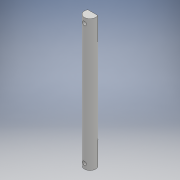
# Autodesk Inventor part: Rear Axle
Saved by Autodesk Inventor 2018 (Build 220112000, 112)
## iProperties
Created: 2018-01-31
Part Number: Rear Axle
Material: Generic
Document SubType Name: Modeling
Designer: alber
Density: 1 g/cm^3
Appearance: Default
Author: alber
Autodesk Inventor part; units mm, degrees
ref_plane "YZ Plane" through (0, 0, 0) normal (1, 0, 0) x (0, 1, 0)
ref_plane "XZ Plane" through (0, 0, 0) normal (0, 1, 0) x (-1, 0, 0)
ref_plane "XY Plane" through (0, 0, 0) normal (0, 0, 1) x (1, 0, 0)
sketch "Sketch1" plane through (0, 0, 0) normal (0, 0, 1) x (1, 0, 0)
  circle A0 centre (0, 0) radius 3.6
  dimension "d0" = 7.2
  constraints: 1 centre point, 1 coincident
  measures "d0" diameter of A0
extrude "Extrusion1" add sketch "Sketch1" along normal mid plane 83.2
sketch "Sketch2" plane through (0, 0, 41.6) normal (0, 0, 1) x (1, 0, 0)
  circle A0 centre (0, 0) radius 3.6 projected
  line L0 (-3.1177, 1.8) -> (3.1177, 1.8)
  dimension "d3" = 1.8
  constraints: 2 end point, 2 point on circle, 1 horizontal
  measures "d3" distance from line of point (0, 0) L0
extrude "Extrusion2" cut sketch "Sketch2" against normal blind 14.4 contours L0 A0 picked at (-0.8728, 2.0235)
sketch "Sketch3" plane through (-3.1177, 1.8, 41.6) normal (0, 1, 0) x (1, 0, 0)
  line L0 (3.1177, 99.84) -> (3.1177, -16.64) projected
  circle A0 centre (3.1177, 3.2) radius 1.2
  line L1 (6.2354, 0) -> (0, 0) projected
  point P0 (3.1177, 41.6)
  dimension "d6" = 3.2
  dimension "d7" = 2.4
  constraints: 1 centre point, 1 point on line
  measures "d6" distance from line of L1 A0.centre
  measures "d7" diameter of A0
extrude "Extrusion3" cut sketch "Sketch3" against normal through all
mirror "Mirror1" about plane through (0, 0, 0) normal (0, 0, 1) of "Extrusion2", "Extrusion3"
sketch "Sketch4" plane through (0, 0, 0) normal (1, 0, 0) x (0, 1, 0)
  line L0 (1.8, 27.2) -> (3.6, 27.2) projected
  line L1 (3.6, -27.2) -> (3.6, 27.2) projected
  line L2 (1.8, 27.2) -> (3.6, 25.4)
  point P0 (0, 0)
  dimension "d10" = 45
  constraints: 2 end point, 1 point on line
  measures "d10" angle of L0 L2
extrude "Extrusion4" cut sketch "Sketch4" along normal through all both and the other way through all
sketch "Sketch5" plane through (0, 0, 41.6) normal (0, 0, 1) x (1, 0, 0)
  line L0 (3.1177, 1.8) -> (-3.1177, 1.8) projected
  arc A0 (-3.1177, 1.8) -> (3.1177, 1.8) centre (0, 0) ccw projected
  line L1 (-5.265, 6.8) -> (5.265, 6.8)
  arc A1 (-5.265, 6.8) -> (5.265, 6.8) centre (0, 0) ccw
  dimension "d13" = 5
  constraints: 2 end point, 2 point on circle, 1 centre point, 1 other
  measures "d13" radial gap between concentric circles of A0 A1
extrude "Extrusion5" [suppressed]
body "Solid1"
